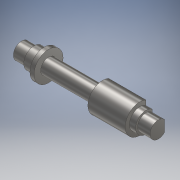
# Autodesk Inventor part: MCP axle
Saved by Autodesk Inventor 2017 (Build 210142000, 142)
## iProperties
Created: 2018-07-30
Part Number: MCP axle
Material: Stainless Steel
Document SubType Name: Modeling
Designer: jakub.tomczynski
Density: 8 g/cm^3
Appearance: Semi-Polished
Author: jakub.tomczynski
Autodesk Inventor part; units mm, degrees
ref_plane "YZ Plane" through (0, 0, 0) normal (1, 0, 0) x (0, 1, 0)
ref_plane "XZ Plane" through (0, 0, 0) normal (0, 1, 0) x (-1, 0, 0)
ref_plane "XY Plane" through (0, 0, 0) normal (0, 0, 1) x (1, 0, 0)
sketch "Sketch1" plane through (0, 0, 0) normal (0, 0, 1) x (1, 0, 0)
  line L0 (-8.25, 0) -> (8.25, 0)
  line L1 (-8.25, 0) -> (-8.25, 1)
  line L2 (-8.25, 1) -> (-6.75, 1)
  line L3 (-6.75, 1) -> (-6.75, 1.25)
  line L4 (-6.75, 1.25) -> (-5.5, 1.25)
  line L5 (-5.5, 1.25) -> (-5.5, 1.25)
  line L6 (-5, 0.95) -> (1.5, 0.95)
  line L7 (1.5, 0.95) -> (1.5, 1.75)
  line L8 (1.5, 1.75) -> (6, 1.75)
  line L9 (6, 1.75) -> (6, 1.25)
  line L10 (6, 1.25) -> (6.75, 1.25)
  line L11 (6.75, 1.25) -> (6.75, 1)
  line L12 (6.75, 1) -> (8.25, 1)
  line L13 (8.25, 1) -> (8.25, 0)
  line L14 (0, 0) -> (0, 3.0708) construction
  line L15 (-5.5, 1.25) -> (-5.5, 1.75)
  line L16 (-5.5, 1.75) -> (-5, 1.75)
  line L17 (-5, 1.75) -> (-5, 0.95)
  dimension "d0" = 2
  dimension "d1" = 16.5
  dimension "d2" = 1.5
  dimension "d3" = 1.5
  dimension "d4" = 2.5
  dimension "d5" = 3.5
  dimension "d6" = 1.9
  dimension "d12" = 7
  dimension "d13" = 0.75
  dimension "d14" = 0.5
  dimension "d16" = 3.5
  dimension "d17" = 1.75
  constraints: 38 end point, 12 perpendicular, 4 point on line, 3 vertical, 1 horizontal, 1 midpoint, 1 other
  measures "d0" diameter of L2 L0
  measures "d1" distance between parallel lines of L13 L1
  measures "d2" distance between parallel lines of L1 L3
  measures "d3" distance between parallel lines of L13 L11
  measures "d4" diameter of L4 L0
  measures "d5" diameter of L8 L0
  measures "d6" diameter of L6 L0
  measures "d12" distance between parallel lines of L7 L5
  measures "d13" distance between parallel lines of L11 L9
  measures "d14" distance between parallel lines of L17 L15
  measures "d16" diameter of L16 L0
  measures "d17" distance between parallel lines of L17 L3
revolve "Revolution1" add sketch "Sketch1" angle 360 about axis through (-8.25, 0, 0) along (1, 0, 0)
sketch "Sketch2" plane through (8.25, 0, 0) normal (1, 0, 0) x (0, 0, -1)
  circle A0 centre (0, 0) radius 1.75 projected
  line L0 (-1.5811, 0.75) -> (1.5811, 0.75)
  dimension "d9" = 0.75
  constraints: 2 end point, 2 point on circle, 1 horizontal
  measures "d9" distance from line of point (0, 0) L0
extrude "Extrusion1" cut sketch "Sketch2" against normal up to surface (6.75 mm away) contours L0 A0 picked at (0, 1.0833)
body "Solid1"
